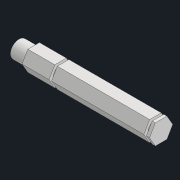
# Autodesk Inventor part: Intermediate Axle
Saved by Autodesk Inventor 2022 (Build 260153000, 153)
## iProperties
Created: 2022-09-07
Part Number: Intermediate Axle
Material: Generic
Document SubType Name: Modeling
Designer: robpl
Density: 1 g/cm^3
Appearance: Default
Author: robpl
Autodesk Inventor part; units mm, degrees
ref_plane "YZ Plane" through (0, 0, 0) normal (1, 0, 0) x (0, 1, 0)
ref_plane "XZ Plane" through (0, 0, 0) normal (0, 1, 0) x (-1, 0, 0)
ref_plane "XY Plane" through (0, 0, 0) normal (0, 0, 1) x (1, 0, 0)
sketch "Sketch1" plane through (0, 0, 0) normal (1, 0, 0) x (0, 1, 0)
  line L0 (4.7625, 2.7496) -> (4.7625, -2.7496)
  line L1 (4.7625, -2.7496) -> (0, -5.4993)
  line L2 (0, -5.4993) -> (-4.7625, -2.7496)
  line L3 (-4.7625, -2.7496) -> (-4.7625, 2.7496)
  line L4 (-4.7625, 2.7496) -> (0, 5.4993)
  line L5 (0, 5.4993) -> (4.7625, 2.7496)
  point P0 (0, 0)
  point P1 (0, 0)
  dimension "d0" = 9.525
  constraints: 12 end point, 1 coincident, 1 vertical, 13 other
  measures "d0" distance between parallel lines of L2 L5
extrude "Extrusion1" add sketch "Sketch1" along normal blind 67.5
sketch "Sketch2" plane through (0, 0, 0) normal (0, 1, 0) x (-1, 0, 0)
  line L0 (-64.8, 13.5) -> (-66, 13.5)
  line L1 (-66, 13.5) -> (-66, 3.5)
  line L2 (-66, 3.5) -> (-64.8, 3.5)
  line L3 (-64.8, 3.5) -> (-64.8, 13.5)
  line L4 (-67.5, 2.7496) -> (-67.5, -2.7496) projected
  line L5 (-21.5, 13.5) -> (-20.3, 13.5)
  line L6 (-20.3, 13.5) -> (-20.3, 3.5)
  line L7 (-20.3, 3.5) -> (-21.5, 3.5)
  line L8 (-21.5, 3.5) -> (-21.5, 13.5)
  line L9 (0, -6.0996) -> (0, 17.3499) projected
  line L10 (13.4, 0) -> (-80.4, 0) projected
  point P0 (0, 0)
  point P1 (0, 0)
  dimension "d3" = 10
  dimension "d4" = 1.2
  dimension "d5" = 1.5
  dimension "d6" = 3.5
  dimension "d7" = 46
  constraints: 16 end point, 4 parallel, 2 equal length, 2 horizontal, 2 perpendicular, 1 coincident, 1 horizontal alignment
  measures "d3" distance of L2.end L0.start
  measures "d4" distance of L0.start L0.end
  measures "d5" distance between parallel lines of L4 L1
  measures "d6" vertical distance of L2.end point (0, 0)
  measures "d7" distance between parallel lines of L8 L4
revolve "Revolution1" cut sketch "Sketch2" angle 360 about axis through (-10, 0, 0) along (1, 0, 0)
sketch "Sketch3" plane through (0, 0, 0) normal (-1, 0, 0) x (0, 0, 1)
  circle A0 centre (0, 0) radius 4
  line L0 (5.4993, 0) -> (2.7496, -4.7625) projected
  line L1 (2.7496, 4.7625) -> (5.4993, 0) projected
  line L2 (-2.7496, 4.7625) -> (2.7496, 4.7625) projected
  line L3 (-5.4993, 0) -> (-2.7496, 4.7625) projected
  line L4 (-2.7496, -4.7625) -> (-5.4993, 0) projected
  line L5 (2.7496, -4.7625) -> (-2.7496, -4.7625) projected
  dimension "d9" = 8
  constraints: 1 centre point, 1 coincident
  measures "d9" diameter of A0
extrude "Extrusion2" cut sketch "Sketch3" against normal blind 7
body "Solid1"
